# Autodesk Inventor part: ICS844071
Saved by Autodesk Inventor 2015 SP1 (Build 190203100, 203)
## iProperties
Created: 2015-06-25
Part Number: ICS844071
Material: Generic
Document SubType Name: Modeling
Designer: Patrick
Density: 1 g/cm^3
Appearance: TSSOP8, ICS844071
Author: Patrick
Autodesk Inventor part; units mm, degrees
ref_plane "YZ Plane" through (0, 0, 0) normal (1, 0, 0) x (0, 1, 0)
ref_plane "XZ Plane" through (0, 0, 0) normal (0, 1, 0) x (-1, 0, 0)
ref_plane "XY Plane" through (0, 0, 0) normal (0, 0, 1) x (1, 0, 0)
sketch "TSSOP8, ICS844071_247" plane through (0, 0, 0) normal (0, 0, 1) x (1, 0, 0)
  line L0 (-4.23, -2.1) -> (-4.23, 2.1)
  line L1 (-4.23, 2.1) -> (3.575, 2.1)
  line L2 (3.575, 2.1) -> (3.575, -2.1)
  line L3 (3.575, -2.1) -> (-4.23, -2.1)
  constraints: 8 end point
extrude "Extrusion1" add sketch "TSSOP8, ICS844071_247" along normal blind 1
body "Solid1"
